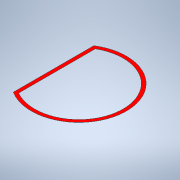
# Autodesk Inventor part: CrowsNestTapeRed
Saved by Autodesk Inventor 2021 (Build 250183000, 183)
## iProperties
Created: 2021-03-04
Part Number: CrowsNestTapeRed
Material: Generic
Document SubType Name: Modeling
Designer: CMurray
Density: 1 g/cm^3
Appearance: Default
Author: CMurray
Autodesk Inventor part; units mm, degrees
ref_plane "YZ Plane" through (0, 0, 0) normal (1, 0, 0) x (0, 1, 0)
ref_plane "XZ Plane" through (0, 0, 0) normal (0, 1, 0) x (-1, 0, 0)
ref_plane "XY Plane" through (0, 0, 0) normal (0, 0, 1) x (1, 0, 0)
sketch "Sketch1" plane through (0, 0, 0) normal (0, 1, 0) x (-1, 0, 0)
  line L0 (378.333, -602.2205) -> (378.333, 602.2205)
  arc A0 (378.333, 602.2205) -> (378.333, -602.2205) centre (0, 0) ccw
  line L1 (327.533, 573.4547) -> (327.533, -573.4547)
  arc A1 (327.533, 573.4547) -> (327.533, -573.4547) centre (0, 0) ccw
  dimension "d3" = 50.8
  constraints: 4 end point, 4 point on circle, 2 centre point, 1 coincident, 1 other
  measures "d3" distance between parallel lines of L0 L1
extrude "Extrusion1" add sketch "Sketch1" along normal blind 1.6002
body "Solid1"
